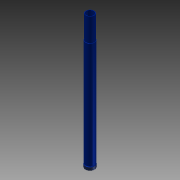
# Autodesk Inventor part: 13_0204_024
Saved by Autodesk Inventor 2012 SP1 (Build 160190100, 190)
## iProperties
Created: 2013-04-03
Part Number: 13_0204_024
Material: Default
Document SubType Name: Modeling
Designer: vogel
Density: 1 g/cm^3
Author: vogel
Autodesk Inventor part; units mm, degrees
ref_plane "YZ Plane" through (0, 0, 0) normal (1, 0, 0) x (0, 1, 0)
ref_plane "XZ Plane" through (0, 0, 0) normal (0, 1, 0) x (-1, 0, 0)
ref_plane "XY Plane" through (0, 0, 0) normal (0, 0, 1) x (1, 0, 0)
sketch "Skizze1" plane through (0, 0, 0) normal (0, 0, 1) x (1, 0, 0)
  circle A0 centre (0, 0) radius 8
  circle A1 centre (0, 0) radius 10.05
  dimension "d0" = 20.1
  dimension "d1" = 2.05
  constraints: 2 centre point, 2 coincident
  measures "d0" diameter of A1
  measures "d1" radial gap between concentric circles of A1 A0
extrude "Extrusion1" add sketch "Skizze1" along normal blind 286
sketch "Skizze2" plane through (0, 0, 286) normal (0, 0, 1) x (1, 0, 0)
  circle A0 centre (0, 0) radius 10.05 projected
  circle A1 centre (0, 0) radius 9.75
  dimension "d4" = 19.5
  constraints: 1 centre point, 1 coincident
  measures "d4" diameter of A1
extrude "Extrusion2" cut sketch "Skizze2" against normal through all
sketch "Skizze3" plane through (0, 0, 0) normal (0, 0, -1) x (-1, 0, 0)
  circle A0 centre (0, 0) radius 9.75 projected
  circle A1 centre (0, 0) radius 8 projected
  circle A2 centre (0, 0) radius 10
  dimension "d7" = 20
  constraints: 1 centre point, 1 coincident
  measures "d7" diameter of A2
extrude "Extrusion3" add sketch "Skizze3" against normal blind 9 contours A2
sketch "Skizze4" plane through (0, 0, 286) normal (0, 0, 1) x (1, 0, 0)
  circle A0 centre (0, 0) radius 9.75 projected
  circle A1 centre (0, 0) radius 8 projected
  circle A2 centre (0, 0) radius 9
  dimension "d10" = 18
  constraints: 1 centre point, 1 coincident
  measures "d10" diameter of A2
extrude "Extrusion4" cut sketch "Skizze4" against normal blind 50 contours A0
sketch "Skizze5" plane through (0, 0, 0) normal (0, 1, 0) x (-1, 0, 0)
  line L0 (-10, 9) -> (10, 9) projected
  line L1 (10, 0) -> (-10, 0) projected
  line L2 (-9.75, 236) -> (9.75, 236) projected
  line L3 (10, 0) -> (10, 9) projected
  line L4 (8, 0) -> (8, 286) projected
  line L5 (9.75, 236) -> (9.75, 9) projected
  line L6 (10, 9) -> (9.25, 9)
  line L7 (9.25, 9) -> (9.25, 7)
  line L8 (9.25, 7) -> (10, 7)
  line L9 (10, 7) -> (10, 9)
  line L10 (14, 0) -> (-14, 0) projected
  line L11 (0, -57.2) -> (0, 343.2) projected
  point P0 (0, 0)
  point P1 (9.9, 9)
  point P2 (-9.9, 9)
  point P3 (9.75, 9)
  dimension "d13" = 2
  dimension "d14" = 18.5
  constraints: 8 end point, 2 parallel, 1 horizontal, 1 perpendicular, 1 other
  measures "d13" distance of L8.end L3.end
  measures "d14" diameter of L7 L11
revolve "Umdrehung1" cut sketch "Skizze5" angle 360 about axis through (0, 0, -10) along (0, 0, 1) contours L0 L3 L8 L7
chamfer "Fase1" distance 0.75 angle 45 1 edges at (10, 0, 7)
thread "Gewinde2" size "M20x1" class "6g" standard "ANSI Metric M Profile" full length
fillet "Rundung1" radius 0.5 1 edges at (-9, 0, 236)
